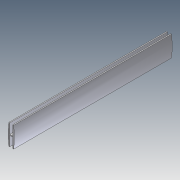
# Autodesk Inventor part: GE-12088-01
Saved by Autodesk Inventor 2012 (Build 160160000, 160)
## iProperties
Created: 2011-11-20
Part Number: GE-12088-01
Document SubType Name: Modeling
Designer: dfoster
Density: 1 g/cm^3
Material: Default
Author: dfoster
Autodesk Inventor part; units mm, degrees
ref_plane "YZ Plane" through (0, 0, 0) normal (1, 0, 0) x (0, 1, 0)
ref_plane "XZ Plane" through (0, 0, 0) normal (0, 1, 0) x (-1, 0, 0)
ref_plane "XY Plane" through (0, 0, 0) normal (0, 0, 1) x (1, 0, 0)
sketch "Sketch1" plane through (0, 0, 0) normal (0, 0, 1) x (1, 0, 0)
  arc A0 (-3.175, 13.2953) -> (-3.175, -13.2953) centre (101.6, 0) ccw
  arc A1 (3.175, -13.2953) -> (3.175, 13.2953) centre (-101.6, 0) ccw
  line L0 (-1.9844, 0.5953) -> (1.9844, 0.5953)
  line L1 (-1.9844, -0.5953) -> (1.9844, -0.5953)
  line L2 (1.9844, 13.2953) -> (1.9844, 0.5953)
  line L3 (1.9844, -0.5953) -> (1.9844, -13.2953)
  line L4 (-1.9844, 13.2953) -> (-1.9844, 0.5953)
  line L5 (-1.9844, -0.5953) -> (-1.9844, -13.2953)
  line L6 (-3.175, 13.2953) -> (-1.9844, 13.2953)
  line L7 (1.9844, 13.2953) -> (3.175, 13.2953)
  line L8 (-3.175, -13.2953) -> (-1.9844, -13.2953)
  line L9 (1.9844, -13.2953) -> (3.175, -13.2953)
  point P0 (0, 0)
  dimension "d4" = 1.9844
  dimension "d5" = 3.9688
  dimension "d6" = 0.5953
  dimension "d7" = 1.1906
  dimension "d8" = 13.2953
  dimension "d9" = 26.5906
  dimension "d10" = 101.6
  dimension "d12" = 1.1906
  constraints: 20 end point, 4 collinear, 4 point on circle, 3 equal length, 2 centre point, 2 horizontal, 1 equal radius, 1 vertical
  measures "d4" distance from line of point (0, 0) L4
  measures "d5" distance between parallel lines of L2 L4
  measures "d6" distance from line of point (0, 0) L0
  measures "d7" distance between parallel lines of L0 L1
  measures "d8" distance from line of point (0, 0) L8
  measures "d9" distance between parallel lines of L6 L8
  measures "d10" distance of point (0, 0) A1.centre
  measures "d12" distance of L2.start L7.end
extrude "Extrusion1" add sketch "Sketch1" along normal blind 203.2
equation "\"d6\" = 0.5 * d7"
equation "\"d12\" = d7"
equation "\"d1\" = 2 * d0"
equation "\"d0\" = 13.295313"
body "Solid1"
